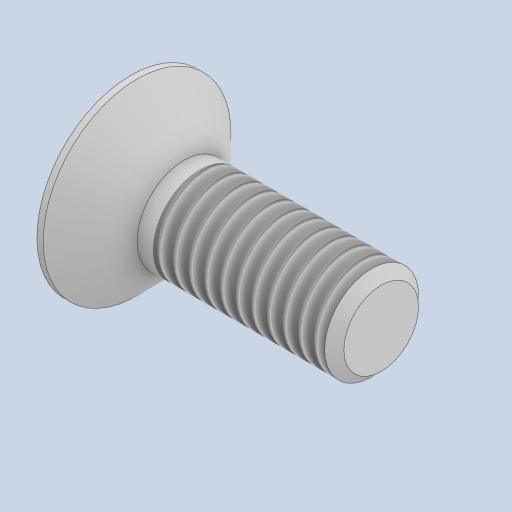
# Autodesk Inventor part: HFBCM3-8
Saved by Autodesk Inventor 2023 (Build 270158000, 158)
## iProperties
Category: PARTsolutions
Company: MISUMI
Created: 2024-12-05
Part Number: HFBCM3-8
Material: Generic
Catalog Web Link: www.cadenas.de
Description: HFBCM, SHFBS, HFBMB-Hexagon Socket Head Cap Screws for Aluminum Frames
Vendor: MISUMI
Document SubType Name: Modeling
Designer: psAdmin
Manufacturer: MISUMI
Mass: 0.0712894 g
Surface Area: 1.32664 cm^2
Volume: 0.0712894 cm^3
Density: 1 g/cm^3
Appearance: PSOLRGB-191-191-191
PSOL_IDENT_0: {$CADENAS_DATA/23d-libs/misumi/metric/38_al_extrusions_blackets/nuts/shfbs.prj},182 {VTYP=3D},{NB=HF
PSOL_IDENT_1: BCM3-8},{LINA=HFBCM3-8},{NN=HFBCM, SHFBS, HFBMB},{DATE=30.07.2021 12:55:02},{GEOMDATE=22.09.2009 00:
PSOL_IDENT_2: 00:00},{VERSION=},{LINEID=10},{WBVAR=MAT,ST,L,SET},{WBNUMERIC=L}  {NB=HFBCM3-8},{LINA=HFBCM3-8},{KT=
PSOL_IDENT_3: DUMMY},{PN=HFBCM3-8},{MAT=HFB},{MATA= 'HFB', 'SCM435(4137 Alloy Steel)(1.7220_34CrMo4)' , 'SHFB'  , '
PSOL_IDENT_4: SUS304(304 Stainless Steel)(1.4301_X5CrNi18-10)' },{ST=CM},{STA= 'CM' , 'Trivalent Chromate Plating'
PSOL_IDENT_5: , 'MB' , 'Trivalent Chromate (Black)' },{M=3},{L=8},{LL=Full Thread},{LLN=5.8},{M1=3},{LA=6,8,10,12
PSOL_IDENT_6: },{NDM=3},{KDM=2.385665},{MP=3X0.5},{A=6},{E=1.7},{B=2.0},{SET=},{SETA='', 'w/o SET1 (Set of 500pcs.
PSOL_IDENT_7: )', '-SET1'  , 'with SET1 (Set of 500pcs.)'},{P=0.50},{COLOR=0.75,0.75,0.75,0.00}
NB: HFBCM3-8
NN: HFBCM, SHFBS, HFBMB
NT: Hexagon Socket Head Cap Screws for Aluminum Frames
NBSYN: $PN.
LINA: HFBCM3-8
CATALOG: Misumi
PN: HFBCM3-8
MAT: 4137 Alloy Steel
ST: Trivalent Chromate Plating
M: 3
L: 8
LL: Full Thread
MP: 3X0.5
A: 6
E: 1.7
B: 2
SET: w/o SET1 (Set of 500pcs.)
SUPPLIER: MISUMI
ARTICLENO: HFBCM3-8
BOMINFO: HFBCM3-8
CREATOR: CADENAS GmbH
Title: HFBCM3-8
Author: Cadenas PARTsolutions
Comments: Hexagon Socket Head Cap Screws for Aluminum Frames
Autodesk Inventor part; units mm, degrees
ref_plane "YZ Plane" through (0, 0, 0) normal (1, 0, 0) x (0, 1, 0)
ref_plane "XZ Plane" through (0, 0, 0) normal (0, 1, 0) x (-1, 0, 0)
ref_plane "XY Plane" through (0, 0, 0) normal (0, 0, 1) x (1, 0, 0)
sketch "Sketch_1" plane through (0, 0, 0) normal (0, 0, 1) x (1, 0, 0)
  line L0 (6.3, 0) -> (0, 0)
  line L1 (-1.7, 0) -> (-1.7, 3)
  line L2 (-1.7, 3) -> (-1.5, 3)
  line L3 (-1.5, 3) -> (0, 1.5)
  line L4 (0, 1.5) -> (5.9935, 1.5)
  line L5 (5.9935, 1.5) -> (6.3, 1.1935)
  line L6 (6.3, 1.1935) -> (6.3, 0)
  line L7 (6.3, 0) -> (-1.7, 0)
  constraints: 16 end point
revolve "Revolution1" add sketch "Sketch_1" angle 360 about axis through (6.3, 0, 0) along (1, 0, 0)
thread "Thread1" size "M3x0.5" class "6g" standard "ISO Metric profile" length 5.4935
sketch "Sketch2" plane through (-1.7, 0, 0) normal (-1, 0, 0) x (0, 0, 1)
  point P0 (0, 0)
hole "Hole1" at (-1.7, 0, 0) direction (1, 0, 0) diameter 2 depth 0.85 tip angle 150
sketch "Sketch_3" plane through (-1.7, 0, 0) normal (1, 0, 0) x (0, 0, -1)
  line L0 (-1, -0.5774) -> (0, -1.1547)
  line L1 (0, -1.1547) -> (1, -0.5774)
  line L2 (1, -0.5774) -> (1, 0.5774)
  line L3 (1, 0.5774) -> (0, 1.1547)
  line L4 (0, 1.1547) -> (-1, 0.5774)
  line L5 (-1, 0.5774) -> (-1, -0.5774)
  constraints: 12 end point
extrude "Extrusion1" cut sketch "Sketch_3" along normal blind 0.85
ref_plane "bolt_to_nut_XY" through (6.3, 0, 0) normal (1, 0, 0) x (0, 0, -1)
ref_plane "bolt_to_nut_YZ" through (6.3, 0, 0) normal (0, 0, -1) x (0, 1, 0)
ref_plane "bolt_to_nut_ZX" through (6.3, 0, 0) normal (0, 1, 0) x (1, 0, 0)
ref_plane "dummy_to_bolt_XY" through (0, 0, 0) normal (1, 0, 0) x (0, 0, -1)
ref_plane "dummy_to_bolt_YZ" through (0, 0, 0) normal (0, 0, -1) x (0, 1, 0)
ref_plane "dummy_to_bolt_ZX" through (0, 0, 0) normal (0, 1, 0) x (1, 0, 0)
body "Solid1"
